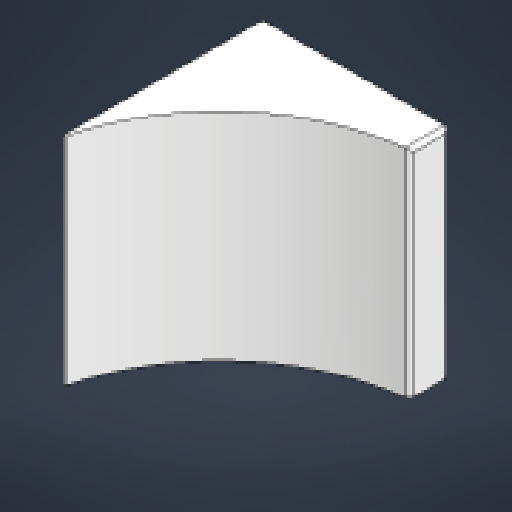
# Autodesk Inventor part: 3DPRINT,KICKER,RAMP
Saved by Autodesk Inventor 2026.1 (Build 301233020, 233B)
## iProperties
Created: 2026-02-08
Part Number: 3DPRINT,KICKER,RAMP
Material: ABS Plastic
Document SubType Name: Modeling
Designer: littl
Density: 0.306529 g/cm^3
Appearance: Smooth - White
Mass: 299.371 g
Surface Area: 889.64 cm^2
Volume: 964.975 cm^3
Author: littl
Autodesk Inventor part; units mm, degrees
ref_plane "YZ Plane" through (0, 0, 0) normal (1, 0, 0) x (0, 1, 0)
ref_plane "XZ Plane" through (0, 0, 0) normal (0, 1, 0) x (-1, 0, 0)
ref_plane "XY Plane" through (0, 0, 0) normal (0, 0, 1) x (1, 0, 0)
sketch "Sketch1" plane through (0, 0, 0) normal (0, 1, 0) x (-1, 0, 0)
  line L0 (175.3437, -172.339) -> (175.3437, 11.811)
  line L1 (175.3437, -172.339) -> (-0.0024, -172.339)
  line L2 (18.465, 67.3862) -> (177.215, 67.3862) projected
  circle A0 centre (195.757, 2.286) radius 14.2875 projected
  circle A1 centre (18.4396, 11.811) radius 11.5 projected
  circle A2 centre (195.757, 2.286) radius 25.4
  arc A3 (38.8187, -143.764) -> (175.3437, 11.811) centre (18.4396, 11.811) ccw
  line L3 (38.8187, -143.764) -> (38.8187, -172.339)
  line L4 (175.3437, -58.039) -> (181.6937, -58.039)
  line L5 (181.6937, -58.039) -> (181.6937, 24.511)
  line L6 (181.6937, 24.511) -> (175.3437, 24.511)
  line L7 (175.3437, 24.511) -> (175.3437, 11.811)
  point P0 (0, 0)
  point P1 (23.4456, -172.339)
  point P2 (181.6937, -0.235)
  point P3 (181.6937, 4.807)
  dimension "d26" = 172.339
  dimension "d53" = 50.8
  dimension "d54" = 28.575
  dimension "d55" = 136.525
  dimension "d56" = 184.15
  dimension "d59" = 6.35
  dimension "d60" = 114.3
  dimension "d61" = 82.55
  constraints: 14 end point, 5 perpendicular, 3 point on line, 2 centre point, 2 coincident, 2 point on circle, 1 collinear, 1 horizontal, 1 horizontal alignment
  measures "d26" distance from line of point (0, 0) L1
  measures "d53" diameter of A2
  measures "d54" distance from line of L1 L3.start
  measures "d55" distance between parallel lines of L0 L3
  measures "d56" distance of L0.start L0.end
  measures "d59" distance of L4.start L4.end
  measures "d60" distance between parallel lines of L1 L4
  measures "d61" distance between parallel lines of L4 L6
extrude "Extrusion1" add sketch "Sketch1" along normal blind 158.75 contours L1 L3 A3 A2 L0 | L0 A2 L5 L4 | A2 A3 L0 | L0 L7 A2 L5 A0 | L7 L6 L5 A2 | A0 L5 picked at (181.6273, 2.5674)
ref_plane "Work Plane1" through (0, 79.375, 0) normal (0, -1, 0) x (1, 0, 0)
fillet "Fillet5" radius 3.175 8 edges at (-38.8187, 79.375, -143.764) (-38.8187, 79.375, -172.339) (-38.8187, 158.75, -158.0515) (-175.3437, 79.375, -172.339) (-175.3437, 79.375, -58.039) (-181.6937, 79.375, -58.039) (-181.6937, 79.375, 24.511) (-175.3437, 79.375, 24.511)
fillet "Fillet5" radius 0.7937 1 edges at (-175.3437, 79.375, 11.811)
sketch "Sketch8" plane through (-181.6937, 0, -54.864) normal (-1, 0, 0) x (0, 0, 1)
  line L0 (79.375, 0) -> (79.375, 158.75) projected
  line L1 (79.375, 95.25) -> (28.575, 95.25)
  line L2 (28.575, 95.25) -> (28.575, 63.5)
  line L3 (28.575, 63.5) -> (79.375, 63.5)
  line L4 (79.375, 63.5) -> (79.375, 95.25)
  point P0 (54.864, 0)
  point P1 (28.575, 79.375)
  point P2 (79.375, 79.375)
  dimension "d62" = 31.75
  dimension "d63" = 50.8
  constraints: 8 end point, 2 midpoint, 2 parallel, 1 horizontal, 1 horizontal alignment, 1 perpendicular, 1 point on line
  measures "d62" distance of L1.end L2.end
  measures "d63" distance of L2.end L3.end
extrude "Extrusion5" cut sketch "Sketch8" against normal through all
fillet "Fillet6" radius 3.175 2 edges at (-176.1706, 63.5, -26.289) (-176.1706, 95.25, -26.289)
body "Solid1"
